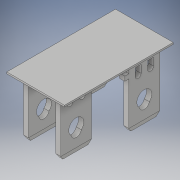
# Autodesk Inventor part: CWSB2F-nonillumin_trmnls
Saved by Autodesk Inventor 2019 (Build 230136000, 136)
## iProperties
Created: 2024-03-12
Part Number: CWSB2F-nonillumin_trmnls
Material: Generic
Catalog Web Link: www.cadenas.de
Description: CWSB - Miniature Power Rockers -nonillumin_trmnls-
Vendor: NKKSWITCHES
Document SubType Name: Modeling
Designer: psAdmin
Manufacturer: NKKSWITCHES
Mass: 0.140159 g
Surface Area: 6.77937 cm^2
Volume: 0.140159 cm^3
Density: 1 g/cm^3
Appearance: PSOLRGB-175-175-175
Category: PARTsolutions
Company: NKKSWITCHES
Title: CWSB2F-nonillumin_trmnls
Author: Cadenas PARTsolutions
PSOL_IDENT_0: {$CADENAS_DATA/23d-libs/nkkswitches/rocker/cw_nonillumin/parts/cwsb_nonillumin_trmnls.prj},241 {VTYP=
PSOL_IDENT_1: 3D},{NB=CWSB2F-nonillumin_trmnls},{LINA=CWSB2F-nonillumin_trmnls},{NN=CWSB - Miniature Power Rockers
PSOL_IDENT_2: -nonillumin_trmnls},{DATE=09.02.2024 16:13:46},{GEOMDATE=06.11.2009 12:09:00},{VERSION=},{LINEID=10
PSOL_IDENT_3: },{WBVAR=PLS,TRMNLS},{WBNUMERIC=}  {NB=CWSB2F-nonillumin_trmnls},{LINA=CWSB2F-nonillumin_trmnls},{KT=
PSOL_IDENT_4: DUMMY},{PN=CWSB2F},{SRS=CWSB},{PLS=2},{TRMNLS=F}
NB: CWSB2F-nonillumin_trmnls
NN: CWSB - Miniature Power Rockers -nonillumin_trmnls
NBSYN: $PN.-nonillumin_trmnls
LINA: CWSB2F-nonillumin_trmnls
CATALOG: NKK Switches
PN: CWSB2F
SRS: CWSB
PLS: 2 - DPST
TRMNLS: F - Quick Connect
SUPPLIER: NKKSWITCHES
ARTICLENO: CWSB2F-nonillumin_trmnls
BOMINFO: CWSB2F-nonillumin_trmnls
CREATOR: CADENAS GmbH
Autodesk Inventor part; units mm, degrees
sketch "Sketch_1" plane through (0, 0.508, 0) normal (0, 1, 0) x (1, 0, 0)
  line L0 (-4.445, 8.382) -> (-4.445, -8.382)
  line L1 (-4.445, -8.382) -> (4.445, -8.382)
  line L2 (4.445, -8.382) -> (4.445, 8.382)
  line L3 (4.445, 8.382) -> (-4.445, 8.382)
  constraints: 8 end point
extrude "Extrusion1" add sketch "Sketch_1" against normal blind 0.254
sketch "Sketch_2" plane through (-2.4892, 0, 0) normal (1, 0, 0) x (0, 0, -1)
  line L0 (-7.3787, -7.62) -> (-6.9342, -8.255)
  line L1 (-6.9342, -8.255) -> (-3.0734, -8.255)
  line L2 (-3.0734, -8.255) -> (-2.6289, -7.62)
  line L3 (-2.6289, -7.62) -> (-2.6289, 0.508)
  line L4 (-2.6289, 0.508) -> (-7.3787, 0.508)
  line L5 (-7.3787, 0.508) -> (-7.3787, -7.62)
  arc A0 (-4.2207, -5.6252) -> (-5.7869, -5.6252) centre (-5.0038, -4.7752) ccw
  arc A1 (-5.7869, -5.6252) -> (-4.2207, -5.6252) centre (-5.0038, -5.461) ccw
  constraints: 12 end point, 4 point on circle, 2 centre point
extrude "Extrusion2" add sketch "Sketch_2" along normal mid plane 0.7874
sketch "Sketch_3" plane through (2.4892, 0, 0) normal (1, 0, 0) x (0, 0, -1)
  line L0 (-7.3787, -7.62) -> (-6.9342, -8.255)
  line L1 (-6.9342, -8.255) -> (-3.0734, -8.255)
  line L2 (-3.0734, -8.255) -> (-2.6289, -7.62)
  line L3 (-2.6289, -7.62) -> (-2.6289, 0.508)
  line L4 (-2.6289, 0.508) -> (-7.3787, 0.508)
  line L5 (-7.3787, 0.508) -> (-7.3787, -7.62)
  arc A0 (-4.2207, -5.6252) -> (-5.7869, -5.6252) centre (-5.0038, -4.7752) ccw
  arc A1 (-5.7869, -5.6252) -> (-4.2207, -5.6252) centre (-5.0038, -5.461) ccw
  constraints: 12 end point, 4 point on circle, 2 centre point
extrude "Extrusion3" add sketch "Sketch_3" along normal mid plane 0.7874
sketch "Sketch_4" plane through (-3.9878, 0, 0) normal (1, 0, 0) x (0, 0, -1)
  line L0 (0.9779, -0.3048) -> (0.9779, -1.016)
  line L1 (0.9779, -1.016) -> (1.6129, -1.016)
  line L2 (1.6129, -1.016) -> (1.6129, -7.62)
  line L3 (1.6129, -7.62) -> (2.0574, -8.255)
  line L4 (2.0574, -8.255) -> (5.9182, -8.255)
  line L5 (5.9182, -8.255) -> (6.3627, -7.62)
  line L6 (6.3627, -7.62) -> (6.3627, 0.508)
  line L7 (6.3627, 0.508) -> (1.6129, 0.508)
  line L8 (1.6129, 0.508) -> (1.6129, -0.3048)
  line L9 (1.6129, -0.3048) -> (0.9779, -0.3048)
  arc A0 (4.7709, -5.6252) -> (3.2047, -5.6252) centre (3.9878, -4.7752) ccw
  arc A1 (3.2047, -5.6252) -> (4.7709, -5.6252) centre (3.9878, -5.461) ccw
  constraints: 20 end point, 4 point on circle, 2 centre point
extrude "Extrusion4" add sketch "Sketch_4" along normal mid plane 0.7874
sketch "Sketch_5" plane through (3.9878, 0, 0) normal (1, 0, 0) x (0, 0, -1)
  line L0 (0.9779, -0.3048) -> (0.9779, -1.016)
  line L1 (0.9779, -1.016) -> (1.6129, -1.016)
  line L2 (1.6129, -1.016) -> (1.6129, -7.62)
  line L3 (1.6129, -7.62) -> (2.0574, -8.255)
  line L4 (2.0574, -8.255) -> (5.9182, -8.255)
  line L5 (5.9182, -8.255) -> (6.3627, -7.62)
  line L6 (6.3627, -7.62) -> (6.3627, 0.508)
  line L7 (6.3627, 0.508) -> (1.6129, 0.508)
  line L8 (1.6129, 0.508) -> (1.6129, -0.3048)
  line L9 (1.6129, -0.3048) -> (0.9779, -0.3048)
  arc A0 (4.7709, -5.6252) -> (3.2047, -5.6252) centre (3.9878, -4.7752) ccw
  arc A1 (3.2047, -5.6252) -> (4.7709, -5.6252) centre (3.9878, -5.461) ccw
  constraints: 20 end point, 4 point on circle, 2 centre point
extrude "Extrusion5" add sketch "Sketch_5" along normal mid plane 0.7874
sketch "Sketch_6" plane through (0, 0, 0) normal (0, 0, 1) x (1, 0, 0)
  line L0 (-5.08, -8.636) -> (5.08, -8.636)
  line L1 (5.08, -8.636) -> (5.08, 0)
  line L2 (5.08, 0) -> (4.3815, 0)
  line L3 (4.3815, 0) -> (4.3815, -7.62)
  line L4 (4.3815, -7.62) -> (4.2545, -8.255)
  line L5 (4.2545, -8.255) -> (3.7211, -8.255)
  line L6 (3.7211, -8.255) -> (3.5941, -7.62)
  line L7 (3.5941, -7.62) -> (3.5941, 0)
  line L8 (3.5941, 0) -> (2.8829, 0)
  line L9 (2.8829, 0) -> (2.8829, -7.62)
  line L10 (2.8829, -7.62) -> (2.7559, -8.255)
  line L11 (2.7559, -8.255) -> (2.2225, -8.255)
  line L12 (2.2225, -8.255) -> (2.0955, -7.62)
  line L13 (2.0955, -7.62) -> (2.0955, 0)
  line L14 (2.0955, 0) -> (-2.0955, 0)
  line L15 (-2.0955, 0) -> (-2.0955, -7.62)
  line L16 (-2.0955, -7.62) -> (-2.2225, -8.255)
  line L17 (-2.2225, -8.255) -> (-2.7559, -8.255)
  line L18 (-2.7559, -8.255) -> (-2.8829, -7.62)
  line L19 (-2.8829, -7.62) -> (-2.8829, 0)
  line L20 (-2.8829, 0) -> (-3.5941, 0)
  line L21 (-3.5941, 0) -> (-3.5941, -7.62)
  line L22 (-3.5941, -7.62) -> (-3.7211, -8.255)
  line L23 (-3.7211, -8.255) -> (-4.2545, -8.255)
  line L24 (-4.2545, -8.255) -> (-4.3815, -7.62)
  line L25 (-4.3815, -7.62) -> (-4.3815, 0)
  line L26 (-4.3815, 0) -> (-5.08, 0)
  line L27 (-5.08, 0) -> (-5.08, -8.636)
  constraints: 56 end point
extrude "Extrusion6" cut sketch "Sketch_6" along normal mid plane 17.78
sketch "Sketch_8" plane through (0, 0, 0) normal (1, 0, 0) x (0, 1, 0)
  line L0 (0, 6.4198) -> (-1.1938, 6.4198)
  arc A0 (-1.1938, 6.4198) -> (-1.1938, 5.5054) centre (-1.1938, 5.9626) ccw
  line L1 (-1.1938, 5.5054) -> (0, 5.5054)
  line L2 (0, 5.5054) -> (0, 6.4198)
  constraints: 6 end point, 2 point on circle, 1 centre point
extrude "Extrusion7" cut sketch "Sketch_8" along normal mid plane 17.78
sketch "Sketch_9" plane through (0, 0, 0) normal (1, 0, 0) x (0, 1, 0)
  line L0 (0, 4.5021) -> (-1.1938, 4.5021)
  arc A0 (-1.1938, 4.5021) -> (-1.1938, 3.5877) centre (-1.1938, 4.0449) ccw
  line L1 (-1.1938, 3.5877) -> (0, 3.5877)
  line L2 (0, 3.5877) -> (0, 4.5021)
  constraints: 6 end point, 2 point on circle, 1 centre point
extrude "Extrusion8" cut sketch "Sketch_9" along normal mid plane 17.78
sketch "Sketch_10" plane through (0, 0, 0) normal (1, 0, 0) x (0, 1, 0)
  line L0 (0, -2.5718) -> (-1.1938, -2.5718)
  arc A0 (-1.1938, -2.5718) -> (-1.1938, -3.4862) centre (-1.1938, -3.029) ccw
  line L1 (-1.1938, -3.4862) -> (0, -3.4862)
  line L2 (0, -3.4862) -> (0, -2.5718)
  constraints: 6 end point, 2 point on circle, 1 centre point
extrude "Extrusion9" cut sketch "Sketch_10" along normal mid plane 17.78
sketch "Sketch_11" plane through (0, 0, 0) normal (1, 0, 0) x (0, 1, 0)
  line L0 (0, -4.4894) -> (-1.1938, -4.4894)
  arc A0 (-1.1938, -4.4894) -> (-1.1938, -5.4039) centre (-1.1938, -4.9466) ccw
  line L1 (-1.1938, -5.4039) -> (0, -5.4039)
  line L2 (0, -5.4039) -> (0, -4.4894)
  constraints: 6 end point, 2 point on circle, 1 centre point
extrude "Extrusion10" cut sketch "Sketch_11" along normal mid plane 17.78
ref_plane "to_body_XY" through (0, 0, 0) normal (0, -1, 0) x (1, 0, 0)
ref_plane "to_body_YZ" through (0, 0, 0) normal (1, 0, 0) x (0, 0, 1)
ref_plane "to_body_ZX" through (0, 0, 0) normal (0, 0, 1) x (0, -1, 0)
body "Solid1"
